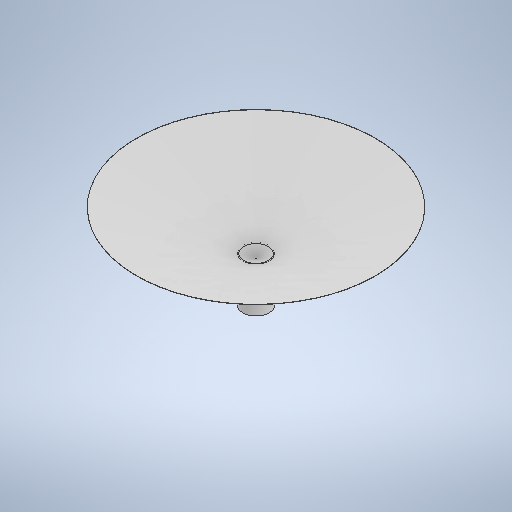
# Autodesk Inventor part: membrane
Saved by Autodesk Inventor 2025.2 (Build 292293000, 293)
## iProperties
Created: 2025-02-21
Part Number: membrane
Material: Generic
Document SubType Name: Modeling
Designer: fiste
Density: 1 g/cm^3
Appearance: Default
Author: fiste
Autodesk Inventor part; units mm, degrees
ref_plane "YZ Plane" through (0, 0, 0) normal (1, 0, 0) x (0, 1, 0)
ref_plane "XZ Plane" through (0, 0, 0) normal (0, 1, 0) x (-1, 0, 0)
ref_plane "XY Plane" through (0, 0, 0) normal (0, 0, 1) x (1, 0, 0)
sketch "Sketch1" plane through (0, 0, 0) normal (0, 1, 0) x (-1, 0, 0)
  line L0 (-0.0702, -39.9737) -> (-106.8222, 0.0263)
  line L1 (-0.0702, -40.1873) -> (-106.8222, -0.1873)
  line L2 (-0.0702, -40.1873) -> (-0.0702, -39.9737)
  line L3 (-106.8222, -0.1873) -> (-106.8222, 0.0263)
  line L4 (0, -48.23) -> (0, 8.069) projected
  dimension "d5" = 114
  dimension "d7" = 0.2
  constraints: 8 end point, 2 vertical, 1 parallel
  measures "d5" distance of L0.start L0.end
  measures "d7" distance between parallel lines of L0 L1
revolve "Revolution1" add sketch "Sketch1" angle 360 about axis through (0, 0, -10) along (0, 0, 1)
sketch "Sketch3" plane through (0, 0, 0) normal (1, 0, 0) x (0, 1, 0)
  line L0 (0.0702, -40.1873) -> (106.8222, -0.1873) projected
  line L1 (11, -36.0919) -> (11, -76.0919)
  line L2 (11, -36.0919) -> (51, -36.0919) construction
  line L3 (11, -76.0919) -> (12, -76.0919)
  line L4 (12, -76.0919) -> (12, -36.0919)
  line L5 (12, -36.0919) -> (11, -36.0919)
  line L6 (0, -91.3155) -> (0, 15.2499) projected
  point P0 (0, 0)
  dimension "d14" = 40
  dimension "d15" = 90
  dimension "d16" = 1
  dimension "d17" = 90
  dimension "d18" = 40
  dimension "d19" = 90
  constraints: 10 end point, 3 perpendicular, 1 horizontal, 1 point on line, 1 vertical
  measures "d14" distance of L1.start L1.end
  measures "d15" angle of L1 L2
  measures "d16" distance of L1.end L3.end
  measures "d17" angle of L3 L1
  measures "d18" distance of L3.end L4.end
  measures "d19" angle of L4 L3
revolve "Revolution3" add sketch "Sketch3" angle 360 about axis through (0, 0, -10) along (0, 0, 1)
